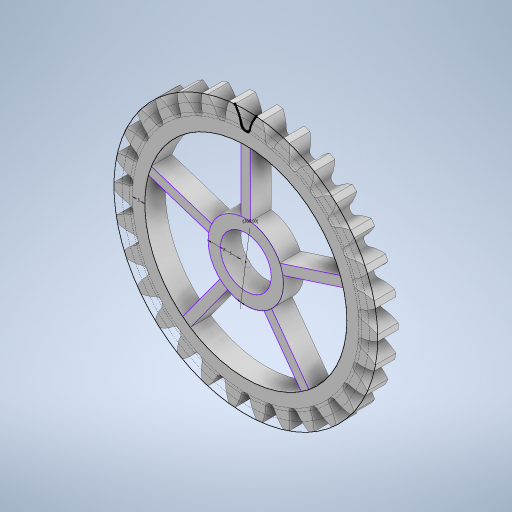
# Autodesk Inventor part: gear_V3
Saved by Autodesk Inventor 2023 (Build 270158000, 158)
## iProperties
Created: 2022-11-24
Part Number: gear_V3
Material: Generic
Document SubType Name: Modeling
Designer: shrey
Density: 1 g/cm^3
Appearance: Default
Author: shrey
Autodesk Inventor part; units mm, degrees
ref_plane "YZ Plane" through (0, 0, 0) normal (1, 0, 0) x (0, 1, 0)
ref_plane "XZ Plane" through (0, 0, 0) normal (0, 1, 0) x (-1, 0, 0)
ref_plane "XY Plane" through (0, 0, 0) normal (0, 0, 1) x (1, 0, 0)
sketch "Sketch1" plane through (0, 0, 0) normal (0, 0, 1) x (1, 0, 0)
  spline S0 degree 3 poles (-2.6107, 31.8933) (-2.5502, 31.7987) (-2.4291, 31.6093) (-2.2562, 31.3199) (-2.0898, 31.0268) (-1.9311, 30.7293) (-1.7805, 30.4277) (-1.6388, 30.1218) (-1.5067, 29.8117) (-1.3854, 29.4971) (-1.2943, 29.2313) (-1.2285, 29.0165) (-1.1831, 28.8541) (-1.1418, 28.6907) (-1.1067, 28.5259) (-1.079, 28.3881) (-1.0493, 28.2797) (-1.0226, 28.1997) (-0.9926, 28.121) (-0.9582, 28.044) (-0.9187, 27.9695) (-0.8741, 27.8979) (-0.8241, 27.83) (-0.7687, 27.7664) (-0.7079, 27.7078) (-0.6416, 27.6557) (-0.5706, 27.6101) (-0.4961, 27.5705) (-0.4173, 27.5402) (-0.336, 27.5176) (-0.2528, 27.5029) (-0.1404, 27.4982) (0, 27.5012) (0.1404, 27.4982) (0.2528, 27.5029) (0.336, 27.5176) (0.4173, 27.5402) (0.4961, 27.5705) (0.5706, 27.6101) (0.6416, 27.6557) (0.7079, 27.7078) (0.7687, 27.7664) (0.8241, 27.83) (0.8741, 27.8979) (0.9187, 27.9695) (0.9582, 28.044) (0.9926, 28.121) (1.0226, 28.1997) (1.0493, 28.2797) (1.079, 28.3881) (1.1067, 28.5259) (1.1418, 28.6907) (1.1831, 28.8541) (1.2285, 29.0165) (1.2943, 29.2313) (1.3854, 29.4971) (1.5067, 29.8117) (1.6388, 30.1218) (1.7805, 30.4277) (1.9311, 30.7293) (2.0898, 31.0268) (2.2562, 31.3199) (2.4291, 31.6093) (2.5502, 31.7987) (2.6107, 31.8933) knots 0 0 0 0 0.033707 0.067415 0.101122 0.134829 0.168536 0.202243 0.235949 0.269656 0.303361 0.320215 0.337069 0.353922 0.370775 0.387627 0.396053 0.40448 0.412906 0.421332 0.429758 0.438185 0.446611 0.455037 0.463464 0.471889 0.48031 0.488735 0.49716 0.505584 0.514009 0.522433 0.539287 0.556141 0.564565 0.57299 0.581413 0.589839 0.598264 0.606685 0.61511 0.623537 0.631963 0.640389 0.648815 0.657242 0.665668 0.674093 0.68252 0.690947 0.707798 0.724651 0.741505 0.758359 0.775212 0.808918 0.842624 0.876331 0.910038 0.943745 0.977452 1.011159 1.044867 1.078574 1.078574 1.078574 1.078574
  circle A0 centre (0, 0) radius 27.5 construction
  circle A1 centre (0, 0) radius 28.1908 construction
  circle A2 centre (0, 0) radius 30 construction
  circle A3 centre (0, 0) radius 32
  circle A4 centre (0, 0) radius 24.5
  circle A5 centre (0, 0) radius 1.16 construction
  circle A6 centre (0, 0) radius 9.16
  line L0 (-1.16, 9.0863) -> (-1.16, 24.4725)
  line L1 (1.16, 9.0863) -> (1.16, 24.4725)
  line L2 (-8.2831, 3.911) -> (-22.9163, 8.6657)
  line L3 (-9, 1.7046) -> (-23.6332, 6.4592)
  line L4 (-6.2792, -6.6691) -> (-15.323, -19.1169)
  line L5 (-4.4023, -8.0328) -> (-13.4461, -20.4805)
  line L6 (4.4023, -8.0328) -> (13.4461, -20.4805)
  line L7 (6.2792, -6.6691) -> (15.323, -19.1169)
  line L8 (9, 1.7046) -> (23.6332, 6.4592)
  line L9 (8.2831, 3.911) -> (22.9163, 8.6657)
  circle A7 centre (0, 0) radius 6.16
  point P0 (-2.4306, 31.6084)
  point P1 (-2.2573, 31.3193)
  point P2 (-2.0911, 31.0261)
  point P3 (-1.9325, 30.7286)
  point P4 (-1.782, 30.427)
  point P5 (-1.6404, 30.1211)
  point P6 (-1.5085, 29.8109)
  point P7 (-1.3874, 29.4964)
  point P8 (-1.2784, 29.1774)
  point P9 (-1.2292, 29.0163)
  point P10 (-1.1838, 28.8539)
  point P11 (-1.1428, 28.6905)
  point P12 (-1.107, 28.5258)
  point P13 (-1.0709, 28.3612)
  point P14 (-1.0486, 28.2799)
  point P15 (-1.0221, 28.1999)
  point P16 (-0.9919, 28.1213)
  point P17 (-0.9573, 28.0444)
  point P18 (-0.9179, 27.97)
  point P19 (-0.8732, 27.8985)
  point P20 (-0.8232, 27.8307)
  point P21 (-0.7678, 27.7672)
  point P22 (-0.707, 27.7089)
  point P23 (-0.6408, 27.6568)
  point P24 (-0.57, 27.6111)
  point P25 (-0.4954, 27.572)
  point P26 (-0.4169, 27.5415)
  point P27 (-0.3357, 27.5189)
  point P28 (-0.2526, 27.5048)
  point P29 (-0.1685, 27.5)
  point P30 (0, 27.5)
  point P31 (0.1685, 27.5)
  point P32 (0.2526, 27.5048)
  point P33 (0.3357, 27.5189)
  point P34 (0.4169, 27.5415)
  point P35 (0.4954, 27.572)
  point P36 (0.57, 27.6111)
  point P37 (0.6408, 27.6568)
  point P38 (0.707, 27.7089)
  point P39 (0.7678, 27.7672)
  point P40 (0.8232, 27.8307)
  point P41 (0.8732, 27.8985)
  point P42 (0.9179, 27.97)
  point P43 (0.9573, 28.0444)
  point P44 (0.9919, 28.1213)
  point P45 (1.0221, 28.1999)
  point P46 (1.0486, 28.2799)
  point P47 (1.0709, 28.3612)
  point P48 (1.107, 28.5258)
  point P49 (1.1428, 28.6905)
  point P50 (1.1838, 28.8539)
  point P51 (1.2292, 29.0163)
  point P52 (1.2784, 29.1774)
  point P53 (1.3874, 29.4964)
  point P54 (1.5085, 29.8109)
  point P55 (1.6404, 30.1211)
  point P56 (1.782, 30.427)
  point P57 (1.9325, 30.7286)
  point P58 (2.0911, 31.0261)
  point P59 (2.2573, 31.3193)
  point P60 (2.4306, 31.6084)
  point P61 (8.2831, 3.911)
  point P62 (9, 1.7046)
  point P63 (6.2792, -6.6691)
  point P64 (4.4023, -8.0328)
  point P65 (-4.4023, -8.0328)
  point P66 (-6.2792, -6.6691)
  point P67 (-9, 1.7046)
  dimension "d2" = 3
  dimension "d4" = 8
  dimension "d7" = 360
  dimension "d16" = 5
  constraints: 20 end point, 8 centre point, 6 point on circle, 2 tangent, 1 coincident, 1 parallel, 1 vertical, 162 other
  measures "d2" radial gap between concentric circles of A0 A4
  measures "d4" radial gap between concentric circles of A5 A6
  measures "d16" radial gap between concentric circles of A5 A7
extrude "Extrusion1" add sketch "Sketch1" against normal blind 5 contours A3 S0 | S0 A3 | A4 L7 A6 L8 | L8 A6 L9 A4 | A4 L6 A6 L7 | L9 A6 L1 A4 | A6 | A4 L5 A6 L6 | L1 A6 L0 A4 | A4 L4 A6 L5 | L0 A6 L2 A4 | A4 L3 A6 L4 | L2 A6 L3 A4 | A7
extrude "Extrusion2" cut sketch "Sketch1" against normal through all contours A3 S0 picked at (-0.1928, 30.4435)
extrude "Extrusion3" cut sketch "Sketch1" against normal through all contours A4 L7 A6 L8 | L9 A6 L1 A4 | A4 L5 A6 L6 | L0 A6 L2 A4 | A4 L3 A6 L4 | A7
pattern_circular "Circular Pattern1" count 30 over 360 about axis through (0, 0, 0) along (0, 0, -1) of "Extrusion2"
equation "\"d0\" = FaceWidth"
equation "\"Module\" = 2"
equation "\"PressureAngle\" = 20deg"
equation "\"UnitProfileClearance\" = 0.25"
equation "\"UnitRoundRadius\" = 0.35"
equation "\"HeadDiameter\" = 64"
equation "\"RootDiameter\" = 55"
equation "\"BaseDiameter\" = 56.38156"
equation "\"FaceWidth\" = 5"
equation "\"HelixAngle\" = 0"
equation "\"UnitCorrection\" = 0"
equation "\"UnitAddendumModification\" = 0"
equation "\"CircularPitch\" = 6.283185"
equation "\"UnitBacklashShift\" = 0"
equation "\"TotalToolShift\" = 0"
equation "\"IsInternal\" = 0"
body "Solid1"
